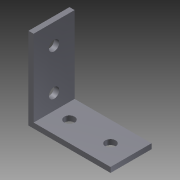
# Autodesk Inventor part: Ad-hoc 2 by 1 angle bracket
Saved by Autodesk Inventor 2011 SP1 (Build 150282100, 282)
## iProperties
Created: 2011-01-12
Part Number: Ad-hoc 2 by 1 angle bracket
Document SubType Name: Modeling
Designer: Christopher
Density: 1 g/cm^3
Author: Christopher
Autodesk Inventor part; units mm, degrees
ref_plane "YZ Plane" through (0, 0, 0) normal (1, 0, 0) x (0, 1, 0)
ref_plane "XZ Plane" through (0, 0, 0) normal (0, 1, 0) x (-1, 0, 0)
ref_plane "XY Plane" through (0, 0, 0) normal (0, 0, 1) x (1, 0, 0)
sketch "Sketch1" plane through (0, 0, 0) normal (0, 0, 1) x (1, 0, 0)
  line L0 (-14.9351, 41.1319) -> (-14.9351, -9.6681)
  line L1 (-14.9351, -9.6681) -> (35.8649, -9.6681)
  line L2 (-11.7601, 41.1319) -> (-11.7601, -6.4931)
  line L3 (-11.7601, -6.4931) -> (35.8649, -6.4931)
  line L4 (35.8649, -9.6681) -> (35.8649, -6.4931)
  line L5 (-14.9351, 41.1319) -> (-11.7601, 41.1319)
  point P0 (0, 0)
  dimension "d0" = 50.8
  dimension "d1" = 50.8
  dimension "d2" = 3.175
  constraints: 12 end point, 4 perpendicular, 1 vertical, 1 other
  measures "d0" distance of L0.start L0.end
  measures "d1" distance of L0.end L1.end
  measures "d2" distance between parallel lines of L1 L3
extrude "Extrusion1" add sketch "Sketch1" against normal blind 25.4
sketch "Sketch2" plane through (-14.9351, -9.6681, 0) normal (-1, 0, 0) x (0, 0, 1)
  line L0 (0, 50.8) -> (-25.4, 50.8) projected
  point P0 (0, 9.6681)
  point P1 (-12.7, 12.7)
  point P2 (-12.7, 38.1)
  dimension "d5" = 12.7
  dimension "d6" = 25.4
  measures "d5" distance from line of L0 point (-12.7, 38.1)
  measures "d6" distance of point (-12.7, 38.1) point (-12.7, 12.7)
sketch "Sketch3" plane through (-14.9351, -9.6681, 0) normal (0, -1, 0) x (1, 0, 0)
  line L0 (50.8, 0) -> (50.8, -25.4) projected
  point P0 (14.9351, 0)
  point P1 (12.7, -12.7)
  point P2 (38.1, -12.7)
  dimension "d7" = 12.7
  dimension "d8" = 25.4
  measures "d7" distance from line of L0 point (38.1, -12.7)
  measures "d8" distance of point (12.7, -12.7) point (38.1, -12.7)
hole "Hole1" at (-14.9351, 28.4319, -12.7) at (-14.9351, 3.0319, -12.7) direction (1, 0, 0) diameter 6.35 depth 25.4 tip angle 118
hole "Hole2" at (-2.2351, -9.6681, -12.7) at (23.1649, -9.6681, -12.7) direction (0, 1, 0) diameter 6.35 depth 25.4 tip angle 118
body "Solid1"
